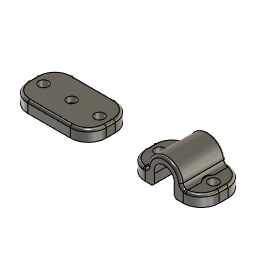
C016 Webcam and Umbilical Mounts (Autodesk Fusion 360 design; units mm, degrees)
Autodesk Fusion 360 part; units mm, degrees
sketch "Sketch1" plane through (0, 0, 0) normal (0, 0, 1) x (1, 0, 0)
  circle A0 centre (0, 0) radius 2.1
  line L0 (17.5, -10) -> (-17.5, -10)
  line L1 (-17.5, -10) -> (-17.5, 10)
  line L2 (-17.5, 10) -> (17.5, 10)
  line L3 (17.5, 10) -> (17.5, -10)
  line L4 (17.5, -10) -> (-17.5, 10) construction
  line L5 (-17.5, -10) -> (17.5, 10) construction
  circle A1 centre (-12.5, 0) radius 2.15
  circle A2 centre (12.5, 0) radius 2.15
  circle A3 centre (0, 0) radius 0.9
  circle A4 centre (-12.5, 0) radius 3.75
  dimension "d1" = 4.2
  dimension "d2" = 35
  dimension "d3" = 20
  dimension "d4" = 4.3
  dimension "d5" = 4.3
  dimension "d6" = 5
  dimension "d7" = 5
  dimension "d8" = 1.8
  dimension "d17" = 7.5
  constraint coincident A0.centre A3.centre
  constraint horizontal L0
  constraint perpendicular L0 L1
  constraint parallel L0 L2
  constraint parallel L1 L3
  constraint coincident L4 A0.centre
  constraint coincident L5 A0.centre
  constraint concentric A0 A3
  constraint concentric A1 A4
  measures "d1" diameter of A0
  measures "d2" distance of L1.end L2.end
  measures "d3" distance of L0.end L1.end
  measures "d4" diameter of A1
  measures "d5" diameter of A2
  measures "d6" distance of L3 A2.centre
  measures "d7" distance of L1 A1.centre
  measures "d8" diameter of A3
  measures "d17" diameter of A4
extrude "Extrude1" add sketch "Sketch1" along normal blind 5 contours L0 L1 L2 L3 | A4 makes body 1
extrude "Extrude2" add sketch "Sketch1" along normal blind 2.4 contours A0 bodies 1
fillet "Fillet1" radius 8 4 edges at (-17.5, 10, 2.5) (-17.5, -10, 2.5) (17.5, 10, 2.5) (17.5, -10, 2.5) on bodies 1
fillet "Fillet2" radius 1 8 edges at (15.1569, -7.6569, 5) (0, -10, 5) (-15.1569, -7.6569, 5) (-17.5, 0, 5) (-15.1569, 7.6569, 5) (0, 10, 5) (15.1569, 7.6569, 5) (17.5, 0, 5) on bodies 1
sketch "Sketch2" plane through (0, 0, 0) normal (0, 1, 0) x (1, 0, 0)
  line L0 (67.9291, -0.0049) -> (67.9291, -5.0049)
  line L1 (34.9291, -5.0049) -> (34.9291, -0.0049)
  arc A0 (43.996, -5.0049) -> (58.8621, -5.0049) centre (51.4291, -6.0049) ccw
  arc A1 (47.0416, -5.0049) -> (55.8674, -5.2624) centre (51.4291, -6.0049) ccw
  line L2 (67.9291, -5.0049) -> (58.8621, -5.0049)
  line L3 (43.996, -5.0049) -> (34.9291, -5.0049)
  line L4 (47.0416, -5.0049) -> (47.0416, -0.0049)
  line L5 (55.8674, -5.2624) -> (55.8674, -0.0049)
  line L6 (34.9291, -0.0049) -> (47.0416, -0.0049)
  line L7 (55.8674, -0.0049) -> (67.9291, -0.0049)
  dimension "d18" = 33
  dimension "d19" = 5
  dimension "d20" = 9
  dimension "d21" = 1
  dimension "d22" = 15
  constraint horizontal L6
  constraint vertical L0
  constraint horizontal L2
  constraint vertical L1
  constraint concentric A0 A1
  constraint coincident A0.start L2
  constraint coincident A1.start L2
  constraint collinear L2 L3
  constraint perpendicular L4 L6
  constraint coincident L5.end L6
  constraint perpendicular L5 L6
  constraint collinear L6 L7
  constraint equal L2 L3
  measures "d18" distance of L1.end L0.start
  measures "d19" distance of L1.end L1.start
  measures "d20" diameter of A1
  measures "d21" distance of A0.centre L2
  measures "d22" diameter of A0
extrude "Extrude3" add sketch "Sketch2" along normal mid plane 20 separate body makes body 2
sketch "Sketch3" plane through (0, 0, 5.0049) normal (0, 0, 1) x (-1, 0, 0)
  line L0 (-43.996, 10) -> (-43.996, -10)
  line L1 (-43.996, -10) -> (-34.9291, -10)
  line L2 (-34.9291, -10) -> (-34.9291, 10)
  line L3 (-34.9291, 10) -> (-43.996, 10)
  line L4 (-67.9291, 10) -> (-67.9291, -10)
  line L5 (-67.9291, -10) -> (-58.8621, -10)
  line L6 (-58.8621, -10) -> (-58.8621, 10)
  line L7 (-58.8621, 10) -> (-67.9291, 10)
  circle A0 centre (-39.4291, 0) radius 2.2
  circle A1 centre (-63.4291, 0) radius 2.2
  circle A2 centre (-63.4291, 0) radius 3.75
  circle A3 centre (-39.4291, 0) radius 3.75
  dimension "d25" = 4.4
  dimension "d26" = 4.4
  dimension "d27" = 4.5
  dimension "d28" = 4.5
  dimension "d37" = 7.5
  dimension "d38" = 7.5
  constraint concentric A1 A2
  constraint concentric A0 A3
  measures "d25" diameter of A0
  measures "d26" diameter of A1
  measures "d27" distance of L2 A0.centre
  measures "d28" distance of L4 A1.centre
  measures "d37" diameter of A2
  measures "d38" diameter of A3
extrude "Extrude4" cut sketch "Sketch3" against normal blind 15.241 contours A0 | A1 bodies 2
fillet "Fillet3" radius 8 4 edges at (67.9291, -10, 2.5049) (34.9291, -10, 2.5049) (34.9291, 10, 2.5049) (67.9291, 10, 2.5049) on bodies 2
fillet "Fillet4" radius 2 2 edges at (43.996, 0, 5.0049) (58.8621, 0, 5.0049) on bodies 2
fillet "Fillet5" radius 1 16 edges at (60.3951, -9.9862, 5.0642) (59.216, -10, 5.8898) (51.4291, -10, 13.5049) (43.6421, -10, 5.8898) (42.463, -9.9862, 5.0642) (36.9467, -7.3114, 5.0049) (34.9291, 0, 5.0049) (36.9467, 7.3114, 5.0049) (42.463, 9.9862, 5.0642) (43.6421, 10, 5.8898) (51.4291, 10, 13.5049) (59.216, 10, 5.8898) (60.3951, 9.9862, 5.0642) (65.9114, 7.3114, 5.0049) (67.9291, 0, 5.0049) (65.9114, -7.3114, 5.0049) on bodies 2
extrude "Extrude5" cut sketch "Sketch3" along normal blind 7.844 contours A2 | A3 bodies 2
chamfer "Chamfer1" distance 1 distance2 1 2 edges at (47.0416, 0, 0.0049) (55.8674, 0, 0.0049) measured on face at (47.0416, -3.3333, 3.3382) measured on face at (57.6546, 0, 0.0049) on bodies 2
equation "d28 = d27"
